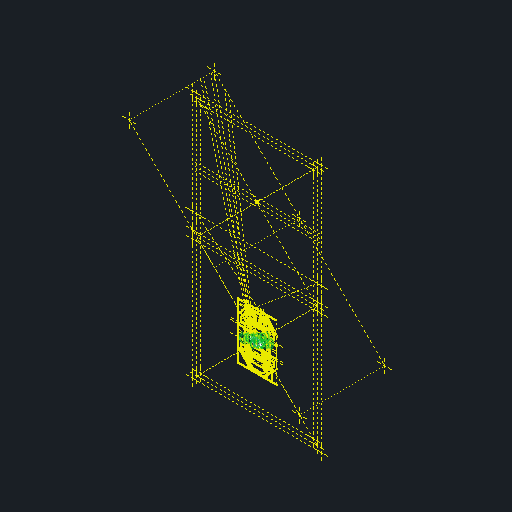
# Autodesk Inventor part: fanmotor-mount-1
Saved by Autodesk Inventor 2023.5 (Build 275446000, 446)
## iProperties
Created: 2025-01-22
Part Number: fanmotor-mount-1
Material: 一般
Document SubType Name: Modeling
Designer: IshiiLabHonda
Density: 1 g/cm^3
Appearance: 既定
Author: IshiiLabHonda
Autodesk Inventor part; units mm, degrees
ref_plane "YZ Plane" through (0, 0, 0) normal (1, 0, 0) x (0, 1, 0)
ref_plane "XZ Plane" through (0, 0, 0) normal (0, 1, 0) x (-1, 0, 0)
ref_plane "XY Plane" through (0, 0, 0) normal (0, 0, 1) x (1, 0, 0)
derived "circuit.ipt"
sketch "スケッチ1" plane through (0, 0, 0) normal (0, 0, 1) x (1, 0, 0)
  line L0 (-90, 90) -> (90, 90) construction
  line L1 (90, 90) -> (90, -90) construction
  line L2 (90, -90) -> (-90, -90) construction
  line L3 (-90, -90) -> (-90, 90) construction
  line L4 (-90, 90) -> (-90, 270) construction
  line L5 (-90, 270) -> (90, 270) construction
  line L6 (90, 270) -> (90, 90) construction
  line L7 (-90, 90) -> (90, -90) construction
  line L8 (90, 90) -> (-90, -90) construction
  line L9 (0, 0) -> (0, 10) construction
  line L10 (0, 0) -> (10, 0) construction
  line L11 (-90, 270) -> (90, 90) construction
  line L12 (-90, 90) -> (90, 270) construction
  line L13 (-96, 276) -> (96, 276) construction
  line L14 (96, 276) -> (96, -96) construction
  line L15 (96, -96) -> (-96, -96) construction
  line L16 (-96, -96) -> (-96, 276) construction
  line L17 (-84, 264) -> (84, 264) construction
  line L18 (84, 264) -> (84, -84) construction
  line L19 (84, -84) -> (-84, -84) construction
  line L20 (-84, -84) -> (-84, 264) construction
  line L21 (-96, 96) -> (96, 96) construction
  line L22 (-96, 84) -> (96, 84) construction
  line L23 (-63.6396, 63.6396) -> (63.6396, 190.9188) construction
  line L24 (63.6396, 190.9188) -> (190.9188, 63.6396) construction
  line L25 (190.9188, 63.6396) -> (63.6396, -63.6396) construction
  line L26 (63.6396, -63.6396) -> (-63.6396, 63.6396) construction
  line L27 (-190.9188, 190.9188) -> (-63.6396, 318.1981) construction
  line L28 (-63.6396, 318.1981) -> (63.6396, 190.9188) construction
  line L29 (-63.6396, 63.6396) -> (-190.9188, 190.9188) construction
  line L30 (-96, 120) -> (96, 120) construction
  line L31 (-96, 186) -> (96, 186) construction
  line L32 (-96, 174) -> (96, 174) construction
  line L33 (-96, 180) -> (96, 180) construction
  point P0 (-63.6396, 318.1981)
  point P1 (-90, 120)
  point P2 (90, 120)
  point P3 (0, 180)
sketch "スケッチ2" plane through (0, 0, 0) normal (0, 0, 1) x (1, 0, 0)
  line L0 (63.6396, 190.9188) -> (190.9188, 63.6396) construction
  line L1 (-63.6396, 318.1981) -> (63.6396, 190.9188) construction
  line L2 (-84, 264) -> (84, 264) construction
  line L3 (-90, 270) -> (90, 270) construction
  line L4 (90, 270) -> (90, 90) construction
  line L5 (-96, 276) -> (96, 276) construction
  line L6 (-90, 90) -> (90, 270) construction
  line L7 (-90, 270) -> (90, 90) construction
  line L8 (-63.6396, 63.6396) -> (63.6396, 190.9188) construction
  line L9 (-96, 120) -> (96, 120) construction
  line L10 (-90, 90) -> (90, 90) construction
  line L11 (-96, 96) -> (96, 96) construction
  line L12 (-96, 84) -> (96, 84) construction
  line L13 (90, -90) -> (-90, -90) construction
  line L14 (0, 0) -> (0, 10) construction
  line L15 (0, 0) -> (10, 0) construction
  line L16 (190.9188, 63.6396) -> (63.6396, -63.6396) construction
  line L17 (63.6396, -63.6396) -> (-63.6396, 63.6396) construction
  line L18 (84, -84) -> (-84, -84) construction
  line L19 (96, -96) -> (-96, -96) construction
  line L20 (-90, 90) -> (-90, 270) construction
  line L21 (-63.6396, 63.6396) -> (-190.9188, 190.9188) construction
  line L22 (-190.9188, 190.9188) -> (-63.6396, 318.1981) construction
  line L23 (96, 276) -> (96, -96) construction
  line L24 (-96, -96) -> (-96, 276) construction
  line L25 (84, 264) -> (84, -84) construction
  line L26 (-84, -84) -> (-84, 264) construction
  line L27 (90, 90) -> (90, -90) construction
  line L28 (-90, 90) -> (90, -90) construction
  line L29 (90, 90) -> (-90, -90) construction
  line L30 (-90, -90) -> (-90, 90) construction
  circle A0 centre (0, 0) radius 16.5 construction
  circle A1 centre (0, 0) radius 10 construction
  line L31 (20, 11.5) -> (28.75, 11.5) construction
  line L32 (28.75, 11.5) -> (28.75, -11.5) construction
  line L33 (28.75, -11.5) -> (20, -11.5) construction
  line L34 (20, -11.5) -> (20, 11.5) construction
  line L35 (20, 11.5) -> (18, 11.5) construction
  line L36 (18, 11.5) -> (18, -11.5) construction
  line L37 (18, -11.5) -> (20, -11.5) construction
  line L38 (18, 1.5) -> (17, 1.5) construction
  line L39 (17, -1.5) -> (18, -1.5) construction
  line L40 (-17, 24) -> (17, 24) construction
  line L41 (17, 24) -> (17, -24) construction
  line L42 (17, -24) -> (-17, -24) construction
  line L43 (-17, -24) -> (-17, 24) construction
  line L44 (-20, 11.5) -> (-28.75, 11.5) construction
  line L45 (-28.75, 11.5) -> (-28.75, -11.5) construction
  line L46 (-28.75, -11.5) -> (-20, -11.5) construction
  line L47 (-20, -11.5) -> (-20, 11.5) construction
  line L48 (-20, 11.5) -> (-18, 11.5) construction
  line L49 (-18, 11.5) -> (-18, -11.5) construction
  line L50 (-18, -11.5) -> (-20, -11.5) construction
  line L51 (-18, 1.5) -> (-17, 1.5) construction
  line L52 (-17, -1.5) -> (-18, -1.5) construction
  line L53 (-14.5, 24) -> (-14.5, -24) construction
  line L54 (14.5, 24) -> (14.5, -24) construction
  line L55 (-10.5, 24) -> (-10.5, 19) construction
  line L56 (-10.5, 19) -> (-14.5, 19) construction
  line L57 (-14.5, 24) -> (-10.5, 19) construction
  line L58 (-10.5, 24) -> (-14.5, 19) construction
  circle A2 centre (-12.5, 21.5) radius 1 construction
  line L59 (10.5, 24) -> (10.5, 19) construction
  line L60 (10.5, 19) -> (14.5, 19) construction
  line L61 (10.5, 24) -> (14.5, 19) construction
  line L62 (10.5, 19) -> (14.5, 24) construction
  circle A3 centre (12.5, 21.5) radius 1 construction
  line L63 (-14.5, -19) -> (-10.5, -19) construction
  line L64 (-10.5, -19) -> (-10.5, -24) construction
  line L65 (10.5, -24) -> (10.5, -19) construction
  line L66 (10.5, -19) -> (14.5, -19) construction
  line L67 (-14.5, -19) -> (-10.5, -24) construction
  line L68 (-10.5, -19) -> (-14.5, -24) construction
  circle A4 centre (-12.5, -21.5) radius 1 construction
  line L69 (10.5, -19) -> (14.5, -24) construction
  line L70 (14.5, -19) -> (10.5, -24) construction
  circle A5 centre (12.5, -21.5) radius 1 construction
  point P0 (90, 120)
  point P1 (-90, 120)
  point P2 (-63.6396, 318.1981)
  point P3 (-12.5, -21.5)
  point P4 (-12.5, 21.5)
sketch "スケッチ3" plane through (0, 0, 0) normal (0, 0, 1) x (1, 0, 0)
  line L0 (63.6396, 190.9188) -> (190.9188, 63.6396) construction
  line L1 (-63.6396, 318.1981) -> (63.6396, 190.9188) construction
  line L2 (-84, 264) -> (84, 264) construction
  line L3 (-90, 270) -> (90, 270) construction
  line L4 (90, 270) -> (90, 90) construction
  line L5 (-96, 276) -> (96, 276) construction
  line L6 (-90, 90) -> (90, 270) construction
  line L7 (-90, 270) -> (90, 90) construction
  line L8 (-63.6396, 63.6396) -> (63.6396, 190.9188) construction
  line L9 (-96, 120) -> (96, 120) construction
  line L10 (-90, 90) -> (90, 90) construction
  line L11 (-96, 96) -> (96, 96) construction
  line L12 (-96, 84) -> (96, 84) construction
  line L13 (90, -90) -> (-90, -90) construction
  line L14 (0, 0) -> (0, 10) construction
  line L15 (0, 0) -> (10, 0) construction
  line L16 (190.9188, 63.6396) -> (63.6396, -63.6396) construction
  line L17 (63.6396, -63.6396) -> (-63.6396, 63.6396) construction
  line L18 (84, -84) -> (-84, -84) construction
  line L19 (96, -96) -> (-96, -96) construction
  line L20 (-90, 90) -> (-90, 270) construction
  line L21 (-63.6396, 63.6396) -> (-190.9188, 190.9188) construction
  line L22 (-190.9188, 190.9188) -> (-63.6396, 318.1981) construction
  line L23 (96, 276) -> (96, -96) construction
  line L24 (-96, -96) -> (-96, 276) construction
  line L25 (84, 264) -> (84, -84) construction
  line L26 (-84, -84) -> (-84, 264) construction
  line L27 (90, 90) -> (90, -90) construction
  line L28 (-90, 90) -> (90, -90) construction
  line L29 (90, 90) -> (-90, -90) construction
  line L30 (-90, -90) -> (-90, 90) construction
  line L31 (-18, 1.5) -> (-17, 1.5) construction
  line L32 (-17, -1.5) -> (-18, -1.5) construction
  line L33 (-20, 11.5) -> (-18, 11.5) construction
  line L34 (-28.75, 11.5) -> (-28.75, -11.5) construction
  line L35 (63.6396, -63.6396) -> (-63.6396, 63.6396) construction
  line L36 (84, -84) -> (-84, -84) construction
  line L37 (-90, -90) -> (-90, 90) construction
  line L38 (96, -96) -> (-96, -96) construction
  line L39 (-90, 90) -> (90, 90) construction
  line L40 (90, -90) -> (-90, -90) construction
  line L41 (90, 90) -> (-90, -90) construction
  line L42 (-90, 90) -> (90, -90) construction
  line L43 (90, 90) -> (90, -90) construction
  line L44 (-28.75, -11.5) -> (-20, -11.5) construction
  line L45 (-20, 11.5) -> (-28.75, 11.5) construction
  line L46 (-18, 11.5) -> (-18, -11.5) construction
  line L47 (-18, -11.5) -> (-20, -11.5) construction
  line L48 (0, 0) -> (0, 10) construction
  line L49 (0, 0) -> (10, 0) construction
  circle A0 centre (0, 0) radius 16.5 construction
  circle A1 centre (0, 0) radius 10 construction
  line L50 (-14.5, 24) -> (-14.5, -24) construction
  line L51 (-17, 24) -> (17, 24) construction
  line L52 (-17, -24) -> (-17, 24) construction
  line L53 (17, -24) -> (-17, -24) construction
  line L54 (-14.5, -19) -> (-10.5, -19) construction
  circle A2 centre (-12.5, -21.5) radius 1 construction
  line L55 (-10.5, -19) -> (-14.5, -24) construction
  line L56 (-14.5, -19) -> (-10.5, -24) construction
  line L57 (-63.6396, 318.1981) -> (63.6396, 190.9188) construction
  line L58 (-84, 264) -> (84, 264) construction
  line L59 (-90, 270) -> (90, 270) construction
  line L60 (90, 270) -> (90, 90) construction
  line L61 (-96, 276) -> (96, 276) construction
  line L62 (-90, 90) -> (90, 270) construction
  line L63 (-90, 270) -> (90, 90) construction
  line L64 (-63.6396, 63.6396) -> (63.6396, 190.9188) construction
  line L65 (-96, 120) -> (96, 120) construction
  line L66 (-96, 96) -> (96, 96) construction
  line L67 (-96, 84) -> (96, 84) construction
  line L68 (84, 264) -> (84, -84) construction
  line L69 (96, 276) -> (96, -96) construction
  line L70 (-96, -96) -> (-96, 276) construction
  line L71 (-84, -84) -> (-84, 264) construction
  line L72 (-63.6396, 63.6396) -> (-190.9188, 190.9188) construction
  line L73 (-90, 90) -> (-90, 270) construction
  line L74 (-190.9188, 190.9188) -> (-63.6396, 318.1981) construction
  line L75 (-20, -11.5) -> (-20, 11.5) construction
  line L76 (10.5, -19) -> (14.5, -19) construction
  line L77 (10.5, -24) -> (10.5, -19) construction
  circle A3 centre (12.5, -21.5) radius 1 construction
  line L78 (10.5, -19) -> (14.5, -24) construction
  line L79 (14.5, -19) -> (10.5, -24) construction
  line L80 (-10.5, -19) -> (-10.5, -24) construction
  line L81 (63.6396, 190.9188) -> (190.9188, 63.6396) construction
  line L82 (190.9188, 63.6396) -> (63.6396, -63.6396) construction
  line L83 (20, 11.5) -> (28.75, 11.5) construction
  line L84 (28.75, 11.5) -> (28.75, -11.5) construction
  line L85 (17, -1.5) -> (18, -1.5) construction
  line L86 (18, -11.5) -> (20, -11.5) construction
  line L87 (28.75, -11.5) -> (20, -11.5) construction
  line L88 (14.5, 24) -> (14.5, -24) construction
  line L89 (17, 24) -> (17, -24) construction
  line L90 (18, 11.5) -> (18, -11.5) construction
  line L91 (20, -11.5) -> (20, 11.5) construction
  line L92 (20, 11.5) -> (18, 11.5) construction
  line L93 (18, 1.5) -> (17, 1.5) construction
  line L94 (-10.5, 24) -> (-10.5, 19) construction
  line L95 (10.5, 19) -> (14.5, 19) construction
  circle A4 centre (12.5, 21.5) radius 1 construction
  line L96 (10.5, 24) -> (14.5, 19) construction
  line L97 (10.5, 19) -> (14.5, 24) construction
  line L98 (10.5, 24) -> (10.5, 19) construction
  line L99 (-10.5, 19) -> (-14.5, 19) construction
  circle A5 centre (-12.5, 21.5) radius 1 construction
  line L100 (-14.5, 24) -> (-10.5, 19) construction
  line L101 (-10.5, 24) -> (-14.5, 19) construction
  line L102 (29.25, 41.5) -> (29.25, -41.5) construction
  line L103 (29.25, -41.5) -> (-29.25, -41.5) construction
  line L104 (-29.25, -41.5) -> (-29.25, 41.5) construction
  line L105 (-29.25, 8.5) -> (-17, 8.5) construction
  line L106 (-17, 8.5) -> (-17, -8.5) construction
  line L107 (-17, -8.5) -> (-29.25, -8.5) construction
  line L108 (29.25, 8.5) -> (17, 8.5) construction
  line L109 (17, 8.5) -> (17, -8.5) construction
  line L110 (17, -8.5) -> (29.25, -8.5) construction
  line L111 (10.0101, 40.6505) -> (14.9894, 36.4724) construction
  line L112 (10.4899, 31.11) -> (12.788, 29.1817) construction
  line L113 (12.788, 29.1817) -> (17.2875, 34.544) construction
  line L114 (10.5581, 32.3582) -> (9.9419, 39.4023) construction
  line L115 (17.2875, 34.544) -> (14.9894, 36.4724) construction
  line L116 (10.4899, 31.11) -> (5.5106, 35.2882) construction
  line L117 (10.5581, 32.3582) -> (6.7279, 35.5721) construction
  line L118 (6.7279, 35.5721) -> (9.9419, 39.4023) construction
  line L119 (5.5106, 35.2882) -> (10.0101, 40.6505) construction
  line L120 (10.0101, 40.6505) -> (10.4899, 31.11) construction
  line L121 (13.7721, 36.1884) -> (10.5581, 32.3582) construction
  line L122 (6.7279, 35.5721) -> (13.7721, 36.1884) construction
  line L123 (5.5106, 35.2882) -> (14.9894, 36.4724) construction
  line L124 (14.9894, 36.4724) -> (10.4899, 31.11) construction
  line L125 (9.9419, 39.4023) -> (13.7721, 36.1884) construction
  line L126 (-7.6191, 6.1457) -> (-8.4873, 11.0698) construction
  line L127 (-2.7087, 12.8503) -> (-1.1893, 4.2332) construction
  line L128 (-3.5633, 11.938) -> (-2.695, 7.014) construction
  line L129 (-7.6191, 6.1457) -> (-3.5633, 11.938) construction
  line L130 (-8.4873, 11.0698) -> (-2.695, 7.014) construction
  line L131 (-9.1099, 11.7216) -> (-2.7087, 12.8503) construction
  line L132 (-1.1893, 4.2332) -> (-7.5905, 3.1045) construction
  line L133 (-7.5905, 3.1045) -> (-9.1099, 11.7216) construction
  line L134 (-63.6396, 318.1981) -> (-5.5912, 9.0419) construction
  line L135 (10.25, 35.8803) -> (-90, 120) construction
  line L136 (-5.5912, 9.0419) -> (-79.4589, 302.3788) construction
  line L137 (-5.5912, 9.0419) -> (-41.5175, 296.076) construction
  line L138 (-9.9419, 39.4023) -> (-6.7279, 35.5721) construction
  line L139 (-10.0101, 40.6505) -> (-5.5106, 35.2882) construction
  line L140 (-14.9894, 36.4724) -> (-10.0101, 40.6505) construction
  line L141 (-5.5106, 35.2882) -> (-14.9894, 36.4724) construction
  line L142 (-13.7721, 36.1884) -> (-6.7279, 35.5721) construction
  line L143 (-13.7721, 36.1884) -> (-9.9419, 39.4023) construction
  line L144 (-14.9894, 36.4724) -> (-17.2875, 34.544) construction
  line L145 (-6.7279, 35.5721) -> (-10.5581, 32.3582) construction
  line L146 (-9.9419, 39.4023) -> (-10.5581, 32.3582) construction
  line L147 (-10.5581, 32.3582) -> (-13.7721, 36.1884) construction
  line L148 (-10.0101, 40.6505) -> (-10.4899, 31.11) construction
  line L149 (-5.5106, 35.2882) -> (-10.4899, 31.11) construction
  line L150 (-10.4899, 31.11) -> (-14.9894, 36.4724) construction
  line L151 (-17.2875, 34.544) -> (-12.788, 29.1817) construction
  line L152 (-12.788, 29.1817) -> (-10.4899, 31.11) construction
  line L153 (-10.25, 35.8803) -> (90, 120) construction
  circle A6 centre (-7.0361, 32.05) radius 0.625 construction
  circle A7 centre (-7.0361, 32.05) radius 0.8 construction
  circle A8 centre (-7.0361, 32.05) radius 1.5 construction
  circle A9 centre (-16.0715, 34.6506) radius 0.625 construction
  circle A10 centre (-16.0715, 34.6506) radius 0.8 construction
  circle A11 centre (-16.0715, 34.6506) radius 1.5 construction
  line L154 (-2.695, 7.014) -> (-7.6191, 6.1457) construction
  line L155 (-7.9812, 5.3203) -> (-1.58, 6.449) construction
  line L156 (-8.0532, 8.6078) -> (-3.1291, 9.476) construction
  line L157 (-4.6361, 3.6254) -> (-5.157, 6.5799) construction
  line L158 (-8.4873, 11.0698) -> (-3.5633, 11.938) construction
  circle A12 centre (7.0361, 32.05) radius 0.625 construction
  circle A13 centre (7.0361, 32.05) radius 0.8
  circle A14 centre (7.0361, 32.05) radius 1.5 construction
  circle A15 centre (16.0715, 34.6506) radius 1.5 construction
  circle A16 centre (16.0715, 34.6506) radius 0.8
  circle A17 centre (16.0715, 34.6506) radius 0.625 construction
  line L159 (-29.25, -41.5) -> (29.25, -41.5)
  line L160 (-29.25, 41.5) -> (29.25, 41.5)
  line L161 (-10.25, 35.8803) -> (-7.0361, 32.05) construction
  line L162 (-29.25, 20.8653) -> (-13.3068, 41.5)
  line L163 (-29.25, -21.1569) -> (-8.9069, -41.5)
  line L164 (29.25, 20.8653) -> (13.3068, 41.5)
  line L165 (29.25, -21.1569) -> (8.9069, -41.5)
  line L166 (25.25, 19.5) -> (25.25, 14.5)
  line L167 (25.25, 14.5) -> (17, 14.5)
  line L168 (-17, 14.5) -> (-25.25, 14.5)
  line L169 (-25.25, 14.5) -> (-25.25, 19.5)
  line L170 (2.7087, 12.8503) -> (1.1893, 4.2332) construction
  line L171 (3.5633, 11.938) -> (2.695, 7.014) construction
  line L172 (8.4873, 11.0698) -> (2.695, 7.014) construction
  line L173 (7.6191, 6.1457) -> (3.5633, 11.938) construction
  line L174 (9.1099, 11.7216) -> (2.7087, 12.8503) construction
  line L175 (7.6191, 6.1457) -> (8.4873, 11.0698) construction
  line L176 (1.1893, 4.2332) -> (7.5905, 3.1045) construction
  line L177 (7.5905, 3.1045) -> (9.1099, 11.7216) construction
  line L178 (2.695, 7.014) -> (7.6191, 6.1457) construction
  line L179 (7.9812, 5.3203) -> (1.58, 6.449) construction
  line L180 (8.4873, 11.0698) -> (3.5633, 11.938) construction
  line L181 (13.5, 24) -> (17, 24)
  line L182 (17, 24) -> (17, 14.5)
  line L183 (-13.5, 24) -> (-17, 24)
  line L184 (-17, 24) -> (-17, 14.5)
  line L185 (-17, -14.5) -> (-25.25, -14.5)
  line L186 (-25.25, -14.5) -> (-25.25, -19.5)
  line L187 (-25.25, -19.5) -> (-7.25, -37.5)
  line L188 (-7.25, -37.5) -> (7.25, -37.5)
  line L189 (7.25, -37.5) -> (25.25, -19.5)
  line L190 (25.25, -19.5) -> (25.25, -14.5)
  line L191 (25.25, -14.5) -> (17, -14.5)
  line L192 (17, -14.5) -> (17, -24)
  line L193 (17, -24) -> (13, -24)
  line L194 (-13, -30) -> (-13, -24)
  line L195 (-13, -24) -> (-17, -24)
  line L196 (-17, -24) -> (-17, -14.5)
  line L197 (-9.1099, 11.7216) -> (-7.5905, 3.1045) construction
  line L198 (-9.4721, 10.8961) -> (-8.6039, 5.9721) construction
  line L199 (-14.3961, 10.0279) -> (-8.6039, 5.9721) construction
  line L200 (-13.5279, 5.1039) -> (-9.4721, 10.8961) construction
  line L201 (-15.5112, 10.5929) -> (-9.1099, 11.7216) construction
  line L202 (-13.5279, 5.1039) -> (-14.3961, 10.0279) construction
  line L203 (-7.5905, 3.1045) -> (-13.9918, 1.9758) construction
  line L204 (-8.6039, 5.9721) -> (-13.5279, 5.1039) construction
  line L205 (-13.962, 7.5659) -> (-9.038, 8.4341) construction
  line L206 (-10.5449, 2.5836) -> (-11.0659, 5.538) construction
  line L207 (-14.3961, 10.0279) -> (-9.4721, 10.8961) construction
  line L208 (9.1099, 11.7216) -> (7.5905, 3.1045) construction
  line L209 (9.4721, 10.8961) -> (8.6039, 5.9721) construction
  line L210 (14.3961, 10.0279) -> (8.6039, 5.9721) construction
  line L211 (13.5279, 5.1039) -> (9.4721, 10.8961) construction
  line L212 (13.5279, 5.1039) -> (14.3961, 10.0279) construction
  line L213 (7.5905, 3.1045) -> (13.9918, 1.9758) construction
  line L214 (13.9918, 1.9758) -> (15.5112, 10.5929) construction
  line L215 (14.3961, 10.0279) -> (9.4721, 10.8961) construction
  line L216 (13.962, 7.5659) -> (9.038, 8.4341) construction
  line L217 (8.6039, 5.9721) -> (13.5279, 5.1039) construction
  line L218 (10.5449, 2.5836) -> (11.0659, 5.538) construction
  line L219 (15.5112, 10.5929) -> (9.1099, 11.7216) construction
  line L220 (-25.25, 19.5) -> (-11.3425, 37.5)
  line L221 (-11.3425, 37.5) -> (11.3425, 37.5)
  line L222 (11.3425, 37.5) -> (25.25, 19.5)
  circle A18 centre (0, 0) radius 4.25 construction
  line L223 (-11.5, 8) -> (-68.7791, 313.0586) construction
  line L224 (-11.5, 8) -> (-84.3887, 297.449) construction
  line L225 (-11.5, 8) -> (-48.4208, 302.9793) construction
  line L226 (-15.5112, 10.5929) -> (-13.9918, 1.9758) construction
  line L227 (-14.3825, 4.1916) -> (-7.9812, 5.3203) construction
  circle A19 centre (-10, -27) radius 1
  circle A20 centre (-10, -27) radius 2
  circle A21 centre (10, -27) radius 1
  circle A22 centre (10, -27) radius 2
  line L228 (-10, -27) -> (10, -27) construction
  line L229 (-13.5, 24) -> (-3, 24)
  line L230 (-13, -30) -> (13, -30)
  line L231 (13, -30) -> (13, -24)
  line L232 (13, -24) -> (13, -24)
  line L233 (-16.1606, 31.2641) -> (-6.1594, 29.9135)
  line L234 (-6.1594, 29.9135) -> (-5.0634, 31.332)
  line L235 (-5.0634, 31.332) -> (-4.8147, 37.5)
  line L236 (16.1606, 31.2641) -> (6.1594, 29.9135)
  line L237 (6.1594, 29.9135) -> (5.0634, 31.332)
  line L238 (5.0634, 31.332) -> (4.8147, 37.5)
  line L239 (-10, -27) -> (-13.875, -30.875) construction
  line L240 (-15.2892, -29.4608) -> (-13, -24)
  line L241 (-12.4608, -32.2892) -> (-7, -30)
  line L242 (-10.5, -19) -> (-10.5, -20.4081)
  line L243 (-10.5, -20.4081) -> (-7.5, -21.5)
  line L244 (-7.5, -21.5) -> (7.5, -21.5)
  line L245 (7.5, -21.5) -> (10.5, -20.4081)
  line L246 (10.5, -20.4081) -> (10.5, -19)
  line L247 (10.5, -19) -> (-10.5, -19)
  line L248 (-10.5, 19) -> (-10.5, 20.4081)
  line L249 (-10.5, 20.4081) -> (-7.5, 21.5)
  line L250 (-7.5, 21.5) -> (7.5, 21.5)
  line L251 (7.5, 21.5) -> (10.5, 20.4081)
  line L252 (10.5, 20.4081) -> (10.5, 19)
  line L253 (10.5, 19) -> (-10.5, 19)
  line L254 (-5.3602, -19) -> (-14.5, -13.3971)
  line L255 (-14.5, -13.3971) -> (-14.5, -15.3971)
  line L256 (0, 0) -> (-9.9301, -16.1985) construction
  line L257 (5.3602, -19) -> (14.5, -13.3971)
  line L258 (14.5, -13.3971) -> (14.5, -15.3971)
  line L259 (-5.3602, 19) -> (-14.5, 13.3971)
  line L260 (-14.5, 13.3971) -> (-14.5, 15.3971)
  line L261 (14.5, 13.3971) -> (14.5, 15.3971)
  line L262 (5.3602, 19) -> (14.5, 13.3971)
  line L263 (-14.5, -15.3971) -> (-10.5, -20.4081)
  line L264 (10.5, -20.4081) -> (14.5, -15.3971)
  line L265 (-14.5, 15.3971) -> (-10.5, 20.4081)
  line L266 (14.5, 15.3971) -> (10.5, 20.4081)
  line L267 (-5.3602, -19) -> (-9.4462, -17.5128)
  line L268 (-9.4462, -17.5128) -> (-14.5, -13.3971)
  line L269 (-10.5, -20.4081) -> (-9.4462, -17.5128) construction
  line L270 (5.3602, -19) -> (9.4462, -17.5128)
  line L271 (9.4462, -17.5128) -> (14.5, -13.3971)
  line L272 (-5.3602, 19) -> (-9.4462, 17.5128)
  line L273 (-9.4462, 17.5128) -> (-14.5, 13.3971)
  line L274 (9.4462, 17.5128) -> (14.5, 13.3971)
  line L275 (5.3602, 19) -> (9.4462, 17.5128)
  line L276 (-3, 24) -> (13.5, 24)
  circle A23 centre (-7, 20) radius 1
  circle A24 centre (-7, 20) radius 2
  circle A25 centre (7, 20) radius 1
  circle A26 centre (7, 20) radius 2
  line L277 (-7, 20) -> (7, 20) construction
  line L278 (-9.4462, 20.7916) -> (-9.4462, 17.5128)
  line L279 (-4.4462, 21.5) -> (-4.4462, 19)
  line L280 (10, -27) -> (13.875, -30.875) construction
  line L281 (15.2892, -29.4608) -> (13, -24)
  line L282 (12.4608, -32.2892) -> (7, -30)
  line L283 (-6.1594, 29.9135) -> (-4.809, 24)
  line L284 (-4.8147, 37.5) -> (-1.7317, 24)
  line L285 (6.1594, 29.9135) -> (4.809, 24)
  line L286 (4.8147, 37.5) -> (1.7317, 24)
  line L287 (9.4462, 20.7916) -> (9.4462, 17.5128)
  line L288 (4.4462, 21.5) -> (4.4462, 19)
  point P0 (90, 120)
  point P1 (90, 120)
  point P2 (11.5, 8)
  point P3 (11.5, 8)
  point P4 (-5.5912, 9.0419)
  point P5 (-5.5912, 9.0419)
  point P6 (6.0926, 30)
  point P7 (5, 19)
sketch "スケッチ4" plane through (0, 0, 0) normal (0, 0, 1) x (1, 0, 0)
  line L0 (0, 0) -> (0, 10) construction
  line L1 (0, 0) -> (10, 0) construction
  line L2 (0, 0) -> (0, 10) construction
  circle A0 centre (0, 0) radius 10 construction
  line L3 (-17, -24) -> (-17, 24) construction
  line L4 (-14.5, 24) -> (-14.5, -24) construction
  line L5 (17, -24) -> (-17, -24) construction
  circle A1 centre (0, 0) radius 16.5 construction
  line L6 (0, 0) -> (10, 0) construction
  line L7 (17, -1.5) -> (18, -1.5) construction
  line L8 (14.5, 24) -> (14.5, -24) construction
  line L9 (17, 24) -> (17, -24) construction
  line L10 (18, 1.5) -> (17, 1.5) construction
  line L11 (18, -11.5) -> (20, -11.5) construction
  line L12 (18, 11.5) -> (18, -11.5) construction
  line L13 (20, -11.5) -> (20, 11.5) construction
  line L14 (20, 11.5) -> (18, 11.5) construction
  line L15 (-18, 11.5) -> (-18, -11.5) construction
  line L16 (-20, -11.5) -> (-20, 11.5) construction
  line L17 (-18, 1.5) -> (-17, 1.5) construction
  line L18 (-17, -1.5) -> (-18, -1.5) construction
  line L19 (-18, -11.5) -> (-20, -11.5) construction
  line L20 (28.75, 11.5) -> (28.75, -11.5) construction
  line L21 (28.75, -11.5) -> (20, -11.5) construction
  line L22 (20, 11.5) -> (28.75, 11.5) construction
  line L23 (-17, 24) -> (17, 24) construction
  line L24 (-20, 11.5) -> (-18, 11.5) construction
  line L25 (-20, 11.5) -> (-28.75, 11.5) construction
  line L26 (-28.75, 11.5) -> (-28.75, -11.5) construction
  line L27 (-28.75, -11.5) -> (-20, -11.5) construction
  line L28 (10.5, -19) -> (14.5, -19) construction
  circle A2 centre (12.5, -21.5) radius 1 construction
  line L29 (10.5, -19) -> (14.5, -24) construction
  line L30 (14.5, -19) -> (10.5, -24) construction
  line L31 (10.5, -24) -> (10.5, -19) construction
  line L32 (-14.5, -19) -> (-10.5, -19) construction
  line L33 (-10.5, -19) -> (-10.5, -24) construction
  line L34 (-14.5, -19) -> (-10.5, -24) construction
  line L35 (-10.5, -19) -> (-14.5, -24) construction
  circle A3 centre (-12.5, -21.5) radius 1 construction
  line L36 (-10.5, 19) -> (-14.5, 19) construction
  circle A4 centre (-12.5, 21.5) radius 1 construction
  line L37 (-14.5, 24) -> (-10.5, 19) construction
  line L38 (-10.5, 24) -> (-14.5, 19) construction
  line L39 (10.5, 19) -> (14.5, 19) construction
  line L40 (10.5, 24) -> (10.5, 19) construction
  circle A5 centre (12.5, 21.5) radius 1 construction
  line L41 (10.5, 24) -> (14.5, 19) construction
  line L42 (10.5, 19) -> (14.5, 24) construction
  line L43 (-10.5, 24) -> (-10.5, 19) construction
  line L44 (0, 0) -> (0, 10) construction
  line L45 (0, 0) -> (10, 0) construction
  line L46 (10.5, -24) -> (10.5, -19) construction
  line L47 (17, -1.5) -> (18, -1.5) construction
  line L48 (18, 1.5) -> (17, 1.5) construction
  line L49 (20, -11.5) -> (20, 11.5) construction
  line L50 (18, 11.5) -> (18, -11.5) construction
  line L51 (28.75, 11.5) -> (28.75, -11.5) construction
  line L52 (-10.5, -19) -> (-10.5, -24) construction
  line L53 (10.5, 19) -> (14.5, 19) construction
  circle A6 centre (12.5, 21.5) radius 1
  line L54 (-17, -1.5) -> (-18, -1.5) construction
  line L55 (14.5, 24) -> (14.5, -24) construction
  line L56 (10.5, 24) -> (14.5, 19) construction
  line L57 (10.5, 19) -> (14.5, 24) construction
  line L58 (17, 24) -> (17, -24) construction
  line L59 (10.5, 24) -> (10.5, 19) construction
  line L60 (-18, 1.5) -> (-17, 1.5) construction
  line L61 (-17, 8.5) -> (-17, -8.5)
  line L62 (-20, 11.5) -> (-18, 11.5) construction
  line L63 (-20, -11.5) -> (-20, 11.5) construction
  line L64 (-29.25, -41.5) -> (-29.25, 41.5)
  line L65 (-28.75, 11.5) -> (-28.75, -11.5) construction
  line L66 (18, -11.5) -> (20, -11.5) construction
  line L67 (10.5, -19) -> (14.5, -19) construction
  line L68 (28.75, -11.5) -> (20, -11.5) construction
  line L69 (10.5, -19) -> (14.5, -24) construction
  line L70 (20, 11.5) -> (18, 11.5) construction
  line L71 (29.25, 8.5) -> (17, 8.5)
  line L72 (20, 11.5) -> (28.75, 11.5) construction
  line L73 (17, 8.5) -> (17, -8.5)
  line L74 (-20, 11.5) -> (-28.75, 11.5) construction
  line L75 (10.0101, 40.6505) -> (14.9894, 36.4724) construction
  line L76 (10.4899, 31.11) -> (12.788, 29.1817) construction
  line L77 (12.788, 29.1817) -> (17.2875, 34.544) construction
  line L78 (10.5581, 32.3582) -> (9.9419, 39.4023) construction
  line L79 (6.7279, 35.5721) -> (9.9419, 39.4023) construction
  line L80 (5.5106, 35.2882) -> (10.0101, 40.6505) construction
  line L81 (10.5581, 32.3582) -> (6.7279, 35.5721) construction
  line L82 (10.4899, 31.11) -> (5.5106, 35.2882) construction
  line L83 (10.0101, 40.6505) -> (10.4899, 31.11) construction
  line L84 (6.7279, 35.5721) -> (13.7721, 36.1884) construction
  line L85 (5.5106, 35.2882) -> (14.9894, 36.4724) construction
  line L86 (9.9419, 39.4023) -> (13.7721, 36.1884) construction
  line L87 (13.7721, 36.1884) -> (10.5581, 32.3582) construction
  line L88 (14.9894, 36.4724) -> (10.4899, 31.11) construction
  line L89 (17.2875, 34.544) -> (14.9894, 36.4724) construction
  circle A7 centre (-12.5, 21.5) radius 1
  line L90 (-10.5, 19) -> (-14.5, 19) construction
  line L91 (-10.5, 24) -> (-10.5, 19) construction
  line L92 (-14.5, 24) -> (-10.5, 19) construction
  line L93 (-10.5, 24) -> (-14.5, 19) construction
  line L94 (-7.6191, 6.1457) -> (-8.4873, 11.0698) construction
  line L95 (-3.5633, 11.938) -> (-2.695, 7.014) construction
  line L96 (-7.6191, 6.1457) -> (-3.5633, 11.938) construction
  line L97 (-8.4873, 11.0698) -> (-2.695, 7.014) construction
  line L98 (-1.1893, 4.2332) -> (-7.5905, 3.1045) construction
  line L99 (-2.7087, 12.8503) -> (-1.1893, 4.2332) construction
  line L100 (-9.1099, 11.7216) -> (-2.7087, 12.8503) construction
  line L101 (-7.5905, 3.1045) -> (-9.1099, 11.7216) construction
  line L102 (-28.75, -11.5) -> (-20, -11.5) construction
  line L103 (-29.25, 8.5) -> (-17, 8.5)
  line L104 (-12.788, 29.1817) -> (-10.4899, 31.11) construction
  circle A8 centre (-16.0715, 34.6506) radius 0.625
  circle A9 centre (-16.0715, 34.6506) radius 0.8 construction
  circle A10 centre (-16.0715, 34.6506) radius 1.5 construction
  line L105 (-17.2875, 34.544) -> (-12.788, 29.1817) construction
  line L106 (-5.5106, 35.2882) -> (-10.4899, 31.11) construction
  line L107 (-6.7279, 35.5721) -> (-10.5581, 32.3582) construction
  line L108 (-5.5106, 35.2882) -> (-14.9894, 36.4724) construction
  line L109 (-13.7721, 36.1884) -> (-6.7279, 35.5721) construction
  line L110 (-10.5581, 32.3582) -> (-13.7721, 36.1884) construction
  line L111 (-14.9894, 36.4724) -> (-17.2875, 34.544) construction
  line L112 (-10.4899, 31.11) -> (-14.9894, 36.4724) construction
  line L113 (-13.7721, 36.1884) -> (-9.9419, 39.4023) construction
  line L114 (-9.9419, 39.4023) -> (-10.5581, 32.3582) construction
  line L115 (-14.9894, 36.4724) -> (-10.0101, 40.6505) construction
  line L116 (-10.0101, 40.6505) -> (-10.4899, 31.11) construction
  line L117 (0, 0) -> (0, 10) construction
  line L118 (0, 0) -> (10, 0) construction
  circle A11 centre (0, 0) radius 10 construction
  line L119 (-14.5, -19) -> (-10.5, -19) construction
  circle A12 centre (0, 0) radius 16.5 construction
  circle A13 centre (12.5, -21.5) radius 1
  line L120 (14.5, -19) -> (10.5, -24) construction
  circle A14 centre (-12.5, -21.5) radius 1
  line L121 (-14.5, -19) -> (-10.5, -24) construction
  line L122 (17, -24) -> (-17, -24) construction
  line L123 (29.25, -41.5) -> (-29.25, -41.5)
  line L124 (-17, -8.5) -> (-29.25, -8.5)
  line L125 (-18, -11.5) -> (-20, -11.5) construction
  line L126 (-18, 11.5) -> (-18, -11.5) construction
  circle A15 centre (-7.0361, 32.05) radius 0.625
  circle A16 centre (-7.0361, 32.05) radius 1.5 construction
  line L127 (-9.9419, 39.4023) -> (-6.7279, 35.5721) construction
  line L128 (-10.0101, 40.6505) -> (-5.5106, 35.2882) construction
  circle A17 centre (-7.0361, 32.05) radius 0.8 construction
  line L129 (-10.5, -19) -> (-14.5, -24) construction
  line L130 (-14.5, 24) -> (-14.5, -24) construction
  line L131 (-17, -24) -> (-17, 24) construction
  line L132 (-17, 24) -> (17, 24) construction
  line L133 (17, -8.5) -> (29.25, -8.5)
  line L134 (-14, 7.5) -> (-14, -7.5)
  line L135 (-14, -7.5) -> (14, -7.5)
  line L136 (14, 7.5) -> (14, -7.5)
  circle A18 centre (-7.25, 0) radius 0.8 construction
  circle A19 centre (0, 0) radius 4.25 construction
  circle A20 centre (0, 0) radius 4.3 construction
  circle A21 centre (0, 0) radius 5.75 construction
  circle A22 centre (-7.25, 0) radius 1.5 construction
  circle A23 centre (7.25, 0) radius 1.5 construction
  circle A24 centre (7.25, 0) radius 0.8 construction
  circle A25 centre (0, 0) radius 1.5
  line L137 (-14, 7.5) -> (14, 7.5)
  line L138 (-14, 7.5) -> (-9.5, 7.5)
  line L139 (-6, 7.5) -> (14, 7.5)
  line L140 (6, -7.5) -> (6, -15.5)
  line L141 (6, -15.5) -> (10, -15.5)
  line L142 (10, -15.5) -> (10, -7.5)
  line L143 (-8, -15.5) -> (10, -15.5)
  line L144 (10, -15.5) -> (10, -21.5)
  line L145 (10, -21.5) -> (-8, -21.5)
  line L146 (-8, -21.5) -> (-8, -15.5)
  line L147 (-8, -18.5) -> (-14, -18.5)
  line L148 (-14, -18.5) -> (-14, -21.5)
  line L149 (-14, -21.5) -> (-8, -21.5)
  line L150 (-8, -21.5) -> (-8, -18.5)
  line L151 (-8, -7.5) -> (6, -7.5)
  line L152 (6, -7.5) -> (6, -9.5)
  line L153 (6, -9.5) -> (-8, -9.5)
  line L154 (-8, -9.5) -> (-8, -7.5)
  line L155 (10, -19.5) -> (14, -19.5)
  line L156 (14, -19.5) -> (14, -21.5)
  line L157 (14, -21.5) -> (10, -21.5)
  line L158 (10, -21.5) -> (10, -19.5)
  line L159 (10, -7.5) -> (14, -7.5)
  line L160 (14, -7.5) -> (14, -10.5)
  line L161 (14, -10.5) -> (10, -10.5)
  line L162 (10, -10.5) -> (10, -7.5)
  line L163 (-14, -21.5) -> (14, -21.5)
  line L164 (14, -21.5) -> (14, -30)
  line L165 (14, -30) -> (-14, -30)
  line L166 (-14, -30) -> (-14, -21.5)
  line L167 (-13, -30) -> (13, -30)
  line L168 (13, -30) -> (13, -24)
  line L169 (13, -24) -> (14, -24)
  line L170 (13, -30) -> (14, -30)
  line L171 (14, -30) -> (14, -24)
  line L172 (-14, -30) -> (-14, -41.5)
  line L173 (-14, -41.5) -> (14, -41.5)
  line L174 (14, -41.5) -> (14, -30)
  line L175 (-29.25, -21.1569) -> (-8.9069, -41.5)
  line L176 (29.25, -21.1569) -> (8.9069, -41.5)
  line L177 (14, -26) -> (22, -26)
  line L178 (22, -26) -> (22, -41.5)
  line L179 (22, -41.5) -> (14, -41.5)
  line L180 (-14, -35.6997) -> (-8.1997, -41.5)
  line L181 (-9.1997, -40.5) -> (9.9069, -40.5)
  line L182 (8.1997, -41.5) -> (22, -27.6997)
  line L183 (-9, 22) -> (9, 22)
  line L184 (9, 22) -> (9, 7.5)
  line L185 (9, 7.5) -> (-9, 7.5)
  line L186 (-9, 7.5) -> (-9, 22)
  circle A26 centre (-7, 20) radius 2
  point P0 (-12.5, -21.5)
  point P1 (-12.5, 21.5)
  point P2 (10.25, 35.8803)
  point P3 (-5.5912, 9.0419)
  point P4 (-10.25, 35.8803)
sketch "スケッチ5" plane through (0, 0, 0) normal (0, 0, 1) x (1, 0, 0)
  circle A0 centre (0, 0) radius 4.25 construction
  circle A1 centre (-7.25, 0) radius 0.8 construction
  circle A2 centre (7.25, 0) radius 0.8 construction
  circle A3 centre (7.25, 0) radius 1.5 projected
  circle A4 centre (-7.25, 0) radius 1.5 projected
  circle A5 centre (0, 0) radius 5.75 projected
  circle A6 centre (0, 0) radius 4.3 projected
  circle A7 centre (-7.25, 0) radius 0.625
  circle A8 centre (7.25, 0) radius 0.625
  line L0 (-8.1293, 1.2152) -> (-3.3707, 4.6584)
  line L1 (0, 0) -> (10, 0) construction
  line L2 (0, 0) -> (0, 10) construction
  line L3 (-8.1293, -1.2152) -> (-3.3707, -4.6584)
  line L4 (8.1293, 1.2152) -> (3.3707, 4.6584)
  line L5 (8.1293, -1.2152) -> (3.3707, -4.6584)
  point P0 (3.3707, -4.6584)
  dimension "d2" = 11.5
  dimension "d3" = 3
  dimension "d1" = 8.6
  dimension "d4" = 1.6
  dimension "d5" = 1.6
  dimension "d6" = 3
  dimension "d7" = 1.25
  dimension "d8" = 1.25
  constraints: 8 end point, 6 symmetric about line, 2 centre point, 2 coincident, 6 other
  measures "d1" diameter of A6
  measures "d4" diameter of A1
  measures "d5" diameter of A2
  measures "d6" diameter of A3
  measures "d7" diameter of A7
  measures "d8" diameter of A8
extrude "押し出し1" add sketch "スケッチ5" along normal blind 3 contours A5 | A6
extrude "押し出し2" add sketch "スケッチ5" along normal blind 1 contours A3 | A3 A5 L4 | L5 A5 A3 | A5 A4 L0 | L3 A4 A5 | A4 | A7 | A8
extrude "押し出し3" cut sketch "スケッチ5" along normal blind 3 contours A6 | A7 | A8
fillet "フィレット1" radius 0.8 3 edges at (-5.75, 0, 1) (5.1207, 2.6154, 1) (5.1207, -2.6154, 1)
